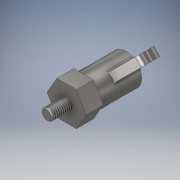
# Autodesk Inventor part: Fusée
Saved by Autodesk Inventor 2019 (Build 230136000, 136)
## iProperties
Created: 2019-07-31
Part Number: Fusée
Material: Acier inoxydable
Document SubType Name: Modeling
Designer: Sébastien DI MERCURIO
Density: 8 g/cm^3
Appearance: Semi-poli
Mass: 12.5786 g
Surface Area: 10.1274 cm^2
Volume: 1.57233 cm^3
Author: Sébastien DI MERCURIO
Autodesk Inventor part; units mm, degrees
ref_plane "XY Plane" through (0, 0, 0) normal (0, 0, 1) x (1, 0, 0)
sketch "Esquisse1" plane through (0, 0, 0) normal (0, 0, 1) x (1, 0, 0)
  circle A0 centre (0, 0) radius 5.5
  dimension "d0" = 11
  constraints: 1 centre point, 1 coincident
  measures "d0" diameter of A0
extrude "Extrusion1" add sketch "Esquisse1" along normal blind 15
ref_plane "Plan de construction1" through (0, 0, 0) normal (0.7071068, -0.7071068, 0) x (0, 0, -1)
sketch "Esquisse3" plane through (0, 0, 0) normal (0.7071068, -0.7071068, 0) x (0, 0, -1)
  circle A0 centre (-9, -7) radius 3
  line L0 (-15, 5.5) -> (-15, -5.5) projected
  line L1 (0, -5.5) -> (0, 5.5) projected
  point P0 (0, 0)
  dimension "d3" = 6
  dimension "d4" = 7
  dimension "d5" = 15
  dimension "d6" = 9
  constraints: 1 centre point
  measures "d3" diameter of A0
  measures "d4" vertical distance of point (0, 0) A0.centre
  measures "d5" distance between parallel lines of L0 L1
  measures "d6" distance from line of A0.centre L1
extrude "Extrusion2" add sketch "Esquisse3" along normal mid plane 11
sketch "Esquisse4" plane through (-8.8388, -1.0607, 9) normal (-0.7071068, 0.7071068, 0) x (-0.7071068, -0.7071068, 0)
  circle A0 centre (0, 0) radius 2
  point P0 (-7, -9)
  dimension "d9" = 4
  constraints: 1 centre point
  measures "d9" diameter of A0
extrude "Extrusion3" cut sketch "Esquisse4" against normal through all
sketch "Esquisse5" plane through (0, 0, 15) normal (0, 0, 1) x (1, 0, 0)
  line L0 (-6.9282, 0) -> (-3.4641, 6)
  line L1 (-3.4641, 6) -> (3.4641, 6)
  line L2 (3.4641, 6) -> (6.9282, 0)
  line L3 (6.9282, 0) -> (3.4641, -6)
  line L4 (3.4641, -6) -> (-3.4641, -6)
  line L5 (-3.4641, -6) -> (-6.9282, 0)
  point P0 (0, 0)
  point P1 (0, 0)
  dimension "d12" = 12
  constraints: 12 end point, 1 coincident, 1 horizontal alignment, 13 other
  measures "d12" distance between parallel lines of L2 L5
extrude "Extrusion4" add sketch "Esquisse5" along normal blind 6
sketch "Esquisse6" plane through (0, 0, 21) normal (0, 0, 1) x (1, 0, 0)
  circle A0 centre (0, 0) radius 2
  dimension "d15" = 4
  constraints: 1 centre point, 1 coincident
  measures "d15" diameter of A0
extrude "Extrusion5" add sketch "Esquisse6" along normal blind 7
thread "Filetage1" size "M4x0.7" class "6g" standard "ANSI Metric M Profile" full length
fillet "Congé1" radius 0.5 1 edges at (-2, 0, 28)
sketch "Esquisse8" plane through (0, 0, 0) normal (0.7071068, -0.7071068, 0) x (0, 0, -1)
  line L0 (0, -5.5) -> (0, 5.5) projected
  line L1 (0, 3.5) -> (-9, 3.5)
  line L2 (-9, 3.5) -> (-9, 17.5)
  line L3 (-9, 17.5) -> (0, 17.5)
  line L4 (0, 17.5) -> (0, 3.5)
  point P0 (0, 0)
  dimension "d21" = 3.5
  dimension "d22" = 14
  dimension "d23" = 9
  constraints: 8 end point, 2 parallel, 1 horizontal, 1 perpendicular, 1 point on line
  measures "d21" distance from line of point (0, 0) L1
  measures "d22" distance of L3.end L1.start
  measures "d23" distance of L2.end L3.end
extrude "Extrusion6" add sketch "Esquisse8" along normal mid plane 3
sketch "Esquisse9" plane through (-1.0607, 1.0607, 0) normal (-0.7071068, 0.7071068, 0) x (-0.7071068, -0.7071068, 0)
  line L0 (-5.2915, 9) -> (-5.2915, 0) projected
  line L1 (-5.2915, 9) -> (-17.5, 6)
  line L2 (-17.5, 9) -> (-17.5, 0) projected
  line L3 (-5.2915, 9) -> (-17.5, 9) projected
  line L4 (-17.5, 9) -> (-5.2915, 9)
  point P0 (0, 0)
  dimension "d26" = 6
  constraints: 4 end point, 1 collinear, 1 point on line
  measures "d26" distance of L2.end L1.end
extrude "Extrusion7" cut sketch "Esquisse9" against normal blind 3
sketch "Esquisse10" plane through (-1.0607, 1.0607, 0) normal (-0.7071068, 0.7071068, 0) x (-0.7071068, -0.7071068, 0)
  circle A0 centre (-14.5, 3) radius 1.5
  line L0 (-17.5, 0) -> (-5.2915, 0) projected
  line L1 (-17.5, 6) -> (-17.5, 0) projected
  point P0 (0, 0)
  dimension "d29" = 3
  dimension "d30" = 3
  dimension "d31" = 3
  constraints: 1 centre point
  measures "d29" distance from line of A0.centre L0
  measures "d30" distance from line of A0.centre L1
  measures "d31" diameter of A0
extrude "Extrusion8" cut sketch "Esquisse10" against normal through all
fillet "Congé2" radius 3 2 edges at (12.3744, 12.3744, 0) (12.3744, 12.3744, 6)
fillet "Congé3" radius 1 2 edges at (2.681, 4.8023, 4.5) (4.8023, 2.681, 4.5)
